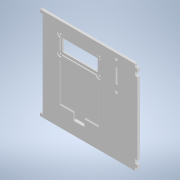
# Autodesk Inventor part: box_front
Saved by Autodesk Inventor 2020 (Build 240168000, 168)
## iProperties
Created: 2020-02-22
Part Number: box_front
Material: Generic
Document SubType Name: Modeling
Designer: Luka
Density: 1 g/cm^3
Appearance: Default
Author: Luka
Autodesk Inventor part; units mm, degrees
ref_plane "YZ Plane" through (0, 0, 0) normal (1, 0, 0) x (0, 1, 0)
sketch "Sketch1" plane through (0, 0, 0) normal (0, 1, 0) x (-1, 0, 0)
  line L0 (200, 200) -> (0, 200)
  line L1 (0, 200) -> (0, 0)
  line L2 (0, 0) -> (200, 0)
  line L3 (200, 0) -> (200, 200)
  dimension "d0" = 200
  dimension "d1" = 200
  constraints: 8 end point, 2 parallel, 1 horizontal, 1 perpendicular
  measures "d0" distance of L2.end L1.end
  measures "d1" distance of L1.end L0.end
extrude "Extrusion1" add sketch "Sketch1" along normal blind 200
shell "Shell1" thickness 5 removed faces 1 at (-66.6667, 200, 133.3333)
sketch "Sketch2" plane through (-200, 0, 200) normal (0, 0, 1) x (1, 0, 0)
  line L0 (155, 170) -> (158.5, 170)
  line L1 (158.5, 170) -> (158.5, 140)
  line L2 (158.5, 140) -> (155, 140)
  line L3 (155, 140) -> (155, 170)
  line L4 (0, 0) -> (0, 200) projected
  line L5 (200, 0) -> (200, 200) projected
  line L6 (0, 200) -> (200, 200) projected
  line L7 (120, 170) -> (40, 170)
  line L8 (40, 170) -> (40, 135)
  line L9 (40, 135) -> (120, 135)
  line L10 (120, 135) -> (120, 170)
  line L11 (40, 125) -> (120, 125)
  line L12 (120, 125) -> (120, 45)
  line L13 (120, 45) -> (40, 45)
  line L14 (40, 45) -> (40, 125)
  line L15 (69, 35) -> (91, 35)
  line L16 (91, 35) -> (91, 31)
  line L17 (91, 31) -> (69, 31)
  line L18 (69, 31) -> (69, 35)
  line L19 (44, 165) -> (116, 165)
  line L20 (116, 165) -> (116, 140)
  line L21 (116, 140) -> (44, 140)
  line L22 (44, 140) -> (44, 165)
  circle A0 centre (40, 170) radius 5
  circle A1 centre (120, 170) radius 5
  circle A2 centre (120, 135) radius 5
  circle A3 centre (40, 135) radius 5
  line L23 (69, 35) -> (91, 35)
  line L24 (91, 35) -> (91, 45)
  line L25 (91, 45) -> (69, 45)
  line L26 (69, 45) -> (69, 35)
  line L27 (200, 0) -> (0, 0) projected
  line L28 (0, 5) -> (200, 5)
  line L29 (195, 5) -> (5, 5) projected
  line L30 (0, 0) -> (0, 200) projected
  line L31 (0, 195) -> (200, 195)
  line L32 (0, 5) -> (0, 0)
  line L33 (200, 0) -> (200, 200) projected
  line L34 (200, 5) -> (200, 0)
  line L35 (0, 195) -> (0, 200)
  line L36 (200, 200) -> (200, 195)
  line L37 (195, 195) -> (195, 189)
  line L38 (195, 189) -> (200, 189)
  line L39 (200, 189) -> (200, 182)
  line L40 (195, 5) -> (195, 200) projected
  line L41 (200, 182) -> (195, 182)
  line L42 (195, 182) -> (195, 174)
  line L43 (195, 174) -> (200, 174)
  line L44 (195, 5) -> (195, 11)
  line L45 (195, 11) -> (200, 11)
  line L46 (200, 11) -> (200, 18)
  line L47 (200, 18) -> (195, 18)
  line L48 (195, 18) -> (195, 26)
  line L49 (195, 26) -> (200, 26)
  line L50 (0, 189) -> (5, 189)
  line L51 (5, 189) -> (5, 11)
  line L52 (5, 11) -> (0, 11)
  point P0 (120, 165)
  point P1 (115, 170)
  point P2 (115, 135)
  point P3 (120, 140)
  point P4 (40, 140)
  point P5 (45, 135)
  point P6 (45, 170)
  point P7 (40, 165)
  point P8 (69, 45)
  point P9 (195, 192)
  point P10 (156.75, 184.188)
  point P11 (156.75, 125.812)
  dimension "COINw" = 3.5
  dimension "COINh" = 30
  dimension "d7" = 155
  dimension "d8" = 41.5
  dimension "d12" = 30
  dimension "d13" = 40
  dimension "LCDw" = 80
  dimension "LCDh" = 35
  dimension "d19" = 22
  dimension "d20" = 4
  dimension "d22" = 29
  dimension "d23" = 10
  dimension "d24" = 10
  dimension "d27" = 72
  dimension "d28" = 25
  dimension "d29" = 4
  dimension "d30" = 4
  dimension "d31" = 5
  dimension "d32" = 5
  dimension "d33" = 10
  dimension "d34" = 10
  dimension "d35" = 10
  dimension "d67" = 10
  dimension "d73" = 5
  dimension "d74" = 6
  dimension "d75" = 7
  dimension "d76" = 8
  dimension "d77" = 6
  dimension "d78" = 7
  dimension "d79" = 8
  dimension "d80" = 5
  dimension "d81" = 6
  dimension "d82" = 6
  dimension "d90" = 14.188
  dimension "d91" = 14.188
  dimension "d92" = 1.75
  dimension "d93" = 1.75
  constraints: 90 end point, 21 point on line, 17 perpendicular, 14 parallel, 9 collinear, 7 horizontal, 4 centre point, 4 coincident, 3 vertical, 1 midpoint
  measures "COINw" distance of L1.end L2.end
  measures "COINh" distance of L0.end L1.end
  measures "d7" distance between parallel lines of L4 L3
  measures "d8" distance between parallel lines of L5 L1
  measures "d12" distance between parallel lines of L6 L0
  measures "d13" distance between parallel lines of L8 L4
  measures "LCDw" distance between parallel lines of L10 L8
  measures "LCDh" distance between parallel lines of L9 L7
  measures "d19" distance of L15.start L15.end
  measures "d20" distance of L15.end L16.end
  measures "d22" distance from line of L13.end L18
  measures "d23" distance between parallel lines of L15 L13
  measures "d24" distance between parallel lines of L11 L9
  measures "d27" distance of L20.end L21.end
  measures "d28" distance of L19.end L20.end
  measures "d29" distance between parallel lines of L8 L22
  measures "d30" distance between parallel lines of L10 L20
  measures "d31" distance between parallel lines of L7 L19
  measures "d32" distance between parallel lines of L9 L21
  measures "d33" diameter of A0
  measures "d34" diameter of A2
  measures "d35" diameter of A3
  measures "d67" diameter of A1
  measures "d73" distance between parallel lines of L31 L6
  measures "d74" distance between parallel lines of L31 L38
  measures "d75" distance between parallel lines of L41 L38
  measures "d76" distance between parallel lines of L43 L41
  measures "d77" distance between parallel lines of L45 L28
  measures "d78" distance between parallel lines of L47 L45
  measures "d79" distance between parallel lines of L49 L47
  measures "d80" distance between parallel lines of L51 L4
  measures "d81" distance between parallel lines of L31 L50
  measures "d82" distance between parallel lines of L28 L52
  measures "d90" distance from line of point (156.75, 184.188) L0
  measures "d91" distance from line of point (156.75, 125.812) L2
  measures "d92" distance from line of L1 point (156.75, 125.812)
  measures "d93" distance from line of L1 point (156.75, 184.188)
extrude "Extrusion2" cut sketch "Sketch2" along normal mid plane 10 contours L0 L1 L2 L3 | L4 L28 L5 L27 | L4 L50 L51 L52 | L28 L40 L45 L5 | L4 L6 L40 L31 | L47 L40 L49 L5 | L40 L6 L5 L31 | L31 L5 L38 L37 | L43 L40 L41 L5 | L15 L16 L17 L18 | L19 L20 L21 L22
sketch "Sketch3" plane through (0, 0, 200) normal (1, 0, 0) x (0, 0, -1)
  line L0 (0, 0) -> (0, 200) projected
  line L1 (0, 80) -> (200, 80)
  line L2 (0, 0) -> (200, 0) projected
  line L3 (195, 5) -> (195, 200) projected
  line L4 (195, 80) -> (195, 0)
  line L5 (95, 80) -> (95, 0)
  line L6 (200, 0) -> (0, 0) projected
  line L7 (5, 5) -> (195, 5) projected
  line L8 (95, 5) -> (195, 5)
  point P0 (195, 198)
  dimension "d16" = 80
  dimension "d44" = 100
  constraints: 8 end point, 8 point on line, 2 perpendicular, 1 collinear, 1 horizontal
  measures "d16" distance between parallel lines of L2 L1
  measures "d44" distance between parallel lines of L3 L5
extrude "Extrusion3" cut sketch "Sketch2" against normal blind 2 contours A0 L8 L7 | L7 L8 A0 | L7 A1 L10 A2 L9 A3 L8 A0 | A1 L10 L7 | L7 L10 A1 | A3 L9 L8 | L8 L9 A3 | A2 L9 L10 | L10 L9 A2 | L11 L12 L13 L14 | L13 L24 L15 L26 | L19 L20 L21 L22
hole "Hole1" at (-160, 170, 200) at (-80, 170, 200) at (-80, 135, 200) at (-160, 135, 200) direction (0, 0, -1) diameter 3.5 depth 5
fillet "Fillet2" radius 3 5 edges at (-160, 85, 198) (-80, 85, 198) (-94.5, 45, 198) (-145.5, 45, 198) (-120, 125, 198)
extrude "Extrusion4" cut sketch "Sketch3" against normal blind 5 contours L1 L3 L7 L5
sketch "Sketch4" plane through (0, 5, 105) normal (0, 0, -1) x (-1, 0, 0)
  circle A0 centre (2.5, 73.5) radius 2.5
  line L0 (0, 0) -> (0, 75) projected
  line L1 (5, 75) -> (5, 0) projected
  circle A1 centre (2.5, 73.5) radius 1
  line L2 (0, 75) -> (5, 75) projected
  line L3 (2.5, 76) -> (2.5, 73.5)
  line L4 (2.5, 73.5) -> (2.5, 71)
  line L5 (2.5, 71) -> (5, 71)
  line L6 (2.5, 76) -> (5, 76)
  line L7 (0, 75) -> (5, 75) projected
  line L8 (5, 76) -> (5, 75)
  point P0 (0, -5)
  point P1 (4.5, 75)
  point P2 (0.5, 75)
  dimension "d47" = 2
  dimension "d48" = 1.5
  constraints: 10 end point, 4 tangent, 2 centre point, 2 perpendicular, 2 point on circle, 2 point on line, 1 coincident, 1 parallel, 1 vertical
  measures "d47" diameter of A1
  measures "d48" distance from line of A0.centre L2
extrude "Extrusion5" add sketch "Sketch4" along normal blind 80 contours L4 A1 L3 L2 A0 | A0 L2 L3 A1 L4
extrude "Extrusion6" cut sketch "Sketch4" along normal blind 60 contours L4 A1 L3 L2 A0 | A0 L2 L3 A1 L4
extrude "Extrusion7" add sketch "Sketch4" along normal blind 40 contours L4 A1 L3 L2 A0 | A0 L2 L3 A1 L4
extrude "Extrusion8" cut sketch "Sketch4" along normal blind 20 contours L4 A1 L3 L2 A0 | A0 L2 L3 A1 L4
fillet "Fillet3" radius 3 2 edges at (-0.5, 80, 75) (-0.5, 80, 35)
fillet "Fillet4" radius 4 2 edges at (-4.5, 80, 75) (-4.5, 80, 35)
extrude "Extrusion9" cut sketch "Sketch4" against normal blind 40 contours L4 L3 A1 | A1 L3 L4
ref_plane "Work Plane1" through (0, 5, 120) normal (0, 0, -1) x (-1, 0, 0)
sketch "Sketch5" plane through (0, 5, 120) normal (0, 0, -1) x (-1, 0, 0)
  circle A0 centre (2.5, 73.5) radius 2.5 projected
  circle A1 centre (2.5, 73.5) radius 1 projected
  line L0 (2.5, 71) -> (5, 71) projected
  line L1 (5, 75) -> (5, 0) projected
  line L2 (5, 71) -> (5, 75)
  line L3 (5, 75) -> (5, 76)
  line L4 (5, 75) -> (5, 195) projected
  line L5 (2.5, 76) -> (5, 76)
  line L6 (2.5, 76) -> (2.5, 71)
  point P0 (0, -5)
  point P1 (5, 193)
  constraints: 8 end point, 1 collinear, 1 point on circle, 1 point on line, 1 tangent, 1 vertical
extrude "Extrusion10" cut sketch "Sketch5" against normal blind 25 contours A0 L6 A1 | L1 L0 A0 | A0 L5 L3 L1 | A1 L6 picked at (4.2027, 74.5258) picked at (3.0499, 73.7078)
ref_plane "Work Plane2" through (-5, 5, 195) normal (0, 0, -1) x (-1, 0, 0)
split "Split1" plane through (-5, 5, 195) removes the side toward (0, 0, -1)
sketch "Sketch6" plane through (-5, 18, 200) normal (0, 1, 0) x (1, 0, 0)
  point P0 (2.5, 2.5)
hole "Hole2" at (-2.5, 18, 197.5) direction (0, -1, 0) diameter 2 depth 7
hole "Hole4" at (-43.25, 184.188, 200) at (-43.25, 125.812, 200) direction (0, 0, -1) diameter 4 depth 5 counterbore diameter 6 counterbore depth 2
sketch "Sketch7" plane through (-5, 189, 200) normal (0, 1, 0) x (1, 0, 0)
  line L0 (5, 5) -> (0, 5) projected
  line L1 (5, 5) -> (5, 0) projected
  point P0 (5, 200)
  point P1 (2.5, 2.5)
  dimension "d101" = 2.5
  dimension "d102" = 2.5
  measures "d101" distance from line of L0 point (2.5, 2.5)
  measures "d102" distance from line of L1 point (2.5, 2.5)
hole "Hole5" at (-2.5, 189, 197.5) direction (0, -1, 0) diameter 2 depth 7
sketch "Sketch8" plane through (-200, 189, 200) normal (0, -1, 0) x (1, 0, 0)
  line L0 (0, -5) -> (5, -5) projected
  line L1 (0, -5) -> (0, 0) projected
  point P0 (200, -200)
  point P1 (2.5, -2.5)
  dimension "d110" = 2.5
  dimension "d111" = 2.5
  measures "d110" distance from line of L0 point (2.5, -2.5)
  measures "d111" distance from line of L1 point (2.5, -2.5)
hole "Hole6" at (-197.5, 189, 197.5) direction (0, 1, 0) diameter 2 depth 6
sketch "Sketch9" plane through (-200, 11, 200) normal (0, 1, 0) x (1, 0, 0)
  line L0 (5, 5) -> (0, 5) projected
  line L1 (0, 0) -> (0, 5) projected
  point P0 (200, 200)
  point P1 (2.5, 2.5)
  dimension "d119" = 2.5
  dimension "d120" = 2.5
  measures "d119" distance from line of L0 point (2.5, 2.5)
  measures "d120" distance from line of L1 point (2.5, 2.5)
hole "Hole7" at (-197.5, 11, 197.5) direction (0, -1, 0) diameter 2 depth 6
equation "\"d45\" = SHELLw"
equation "\"SHELLw\" = 5"
body "Solid1"
